Autodesk Fusion 360 part; units mm, degrees
note: some values were not read from the file. Chosen so that the rebuilt part matches the saved one: which bodies a step acts on. Set by a fixed rule: which sketch regions a step uses.
(part 4 of 6)
sketch "Sketch81" plane through (0, 0, 40) normal (0, 0, 1) x (-1, 0, 0)
  line L0 (-4, -129.3333) -> (-4, -109.2593)
  line L1 (-4, -109.2593) -> (-0.5, -109.2593)
  line L2 (-0.5, -109.2593) -> (-0.5, -90.7407)
  line L3 (-0.5, -90.7407) -> (-4, -90.7407)
  line L4 (-4, -90.7407) -> (-4, -70.6667)
  line L5 (-4, -70.6667) -> (-24.0741, -70.6667)
  line L6 (-24.0741, -70.6667) -> (-24.0741, -67.1667)
  line L7 (-24.0741, -67.1667) -> (-42.5926, -67.1667)
  line L8 (-42.5926, -67.1667) -> (-42.5926, -70.6667)
  line L9 (-42.5926, -70.6667) -> (-62.6667, -70.6667)
  line L10 (-62.6667, -70.6667) -> (-62.6667, -90.7407)
  line L11 (-62.6667, -90.7407) -> (-66.1667, -90.7407)
  line L12 (-66.1667, -90.7407) -> (-66.1667, -109.2593)
  line L13 (-66.1667, -109.2593) -> (-62.6667, -109.2593)
  line L14 (-62.6667, -109.2593) -> (-62.6667, -129.3333)
  line L15 (-62.6667, -129.3333) -> (-42.5926, -129.3333)
  line L16 (-42.5926, -129.3333) -> (-42.5926, -132.8333)
  line L17 (-42.5926, -132.8333) -> (-24.0741, -132.8333)
  line L18 (-24.0741, -132.8333) -> (-24.0741, -129.3333)
  line L19 (-24.0741, -129.3333) -> (-4, -129.3333)
  line L20 (-4, -129.3333) -> (-24.0741, -129.3333)
  line L21 (-24.0741, -129.3333) -> (-24.0741, -128.3333)
  line L22 (-24.0741, -128.3333) -> (-4, -128.3333)
  line L23 (-4, -128.3333) -> (-4, -129.3333)
  line L24 (-4, -129.3333) -> (-5, -129.3333)
  line L25 (-5, -129.3333) -> (-5, -109.2593)
  line L26 (-5, -109.2593) -> (-4, -109.2593)
  line L27 (-4, -109.2593) -> (-4, -129.3333)
  line L28 (-4, -70.6667) -> (-5, -70.6667)
  line L29 (-5, -70.6667) -> (-5, -90.7407)
  line L30 (-5, -90.7407) -> (-4, -90.7407)
  line L31 (-4, -90.7407) -> (-4, -70.6667)
  line L32 (-4, -70.6667) -> (-24.0741, -70.6667)
  line L33 (-24.0741, -70.6667) -> (-24.0741, -71.6667)
  line L34 (-24.0741, -71.6667) -> (-4, -71.6667)
  line L35 (-4, -71.6667) -> (-4, -70.6667)
  line L36 (-62.6667, -70.6667) -> (-42.5926, -70.6667)
  line L37 (-42.5926, -70.6667) -> (-42.5926, -71.6667)
  line L38 (-42.5926, -71.6667) -> (-62.6667, -71.6667)
  line L39 (-62.6667, -71.6667) -> (-62.6667, -70.6667)
  line L40 (-62.6667, -70.6667) -> (-61.6667, -70.6667)
  line L41 (-61.6667, -70.6667) -> (-61.6667, -90.7407)
  line L42 (-61.6667, -90.7407) -> (-62.6667, -90.7407)
  line L43 (-62.6667, -90.7407) -> (-62.6667, -70.6667)
  line L44 (-62.6667, -129.3333) -> (-61.6667, -129.3333)
  line L45 (-61.6667, -129.3333) -> (-61.6667, -109.2593)
  line L46 (-61.6667, -109.2593) -> (-62.6667, -109.2593)
  line L47 (-62.6667, -109.2593) -> (-62.6667, -129.3333)
  line L48 (-62.6667, -129.3333) -> (-42.5926, -129.3333)
  line L49 (-42.5926, -129.3333) -> (-42.5926, -128.3333)
  line L50 (-42.5926, -128.3333) -> (-62.6667, -128.3333)
  line L51 (-62.6667, -128.3333) -> (-62.6667, -129.3333)
  dimension "d549" = 1
  dimension "d550" = 1
  dimension "d551" = 1
  dimension "d552" = 1
  dimension "d553" = 1
  dimension "d554" = 1
  dimension "d555" = 1
  dimension "d556" = 1
  dimension "d557" = 20.0741
  dimension "d558" = 20.0741
  dimension "d559" = 20.0741
  dimension "d560" = 20.0741
  dimension "d561" = 20.0741
  dimension "d562" = 20.0741
  dimension "d563" = 20.0741
  dimension "d564" = 20.0741
  constraint horizontal L20
  constraint vertical L21
  constraint horizontal L22
  constraint vertical L23
  constraint coincident L0.start L19.end
  constraint horizontal L24
  constraint vertical L25
  constraint horizontal L26
  constraint vertical L27
  constraint horizontal L28
  constraint vertical L29
  constraint horizontal L30
  constraint vertical L31
  constraint coincident L4.end L5.start
  constraint horizontal L32
  constraint vertical L33
  constraint horizontal L34
  constraint vertical L35
  constraint horizontal L36
  constraint vertical L37
  constraint horizontal L38
  constraint vertical L39
  constraint coincident L9.end L10.start
  constraint horizontal L40
  constraint vertical L41
  constraint horizontal L42
  constraint vertical L43
  constraint horizontal L44
  constraint vertical L45
  constraint horizontal L46
  constraint vertical L47
  constraint coincident L14.end L15.start
  constraint horizontal L48
  constraint vertical L49
  constraint horizontal L50
  constraint vertical L51
  measures "d549" distance of L18.end L21.end
  measures "d550" distance of L15.end L49.end
  measures "d551" distance of L45.end L13.end
  measures "d552" distance of L9.end L40.end
  measures "d553" distance of L8.end L37.end
  measures "d554" distance of L5.end L33.end
  measures "d555" distance of L29.end L3.end
  measures "d556" distance of L25.end L0.end
  measures "d557" distance of L9.end L10.end
  measures "d558" distance of L14.end L13.end
  measures "d559" distance of L24.end L25.end
  measures "d560" distance of L28.end L29.end
  measures "d561" distance of L4.end L5.end
  measures "d562" distance of L9.end L8.end
  measures "d563" distance of L49.end L50.end
  measures "d564" distance of L21.end L22.end
extrude "Extrude50" cut sketch "Sketch81" against normal blind 4 contours L0 L19 L20 L22 L23 L24 L25 L27 | L0 L22 L25 L26 L27 | L19 L20 L21 L22 L25 | L4 L29 L30 L31 L34 | L15 L45 L48 L49 L50 | L4 L5 L28 L29 L31 L32 L34 L35 | L14 L15 L44 L45 L47 L48 L50 L51 | L5 L29 L32 L33 L34 | L14 L45 L46 L47 L50 | L9 L36 L37 L38 L41 | L10 L38 L41 L42 L43 | L9 L10 L36 L38 L39 L40 L41 L43 bodies 16
sketch "Sketch82" plane through (0, 0, 40) normal (0, 0, 1) x (-1, 0, 0)
  line L0 (-129.3333, -129.3333) -> (-109.2593, -129.3333)
  line L1 (-109.2593, -129.3333) -> (-109.2593, -132.8333)
  line L2 (-109.2593, -132.8333) -> (-90.7407, -132.8333)
  line L3 (-90.7407, -132.8333) -> (-90.7407, -129.3333)
  line L4 (-90.7407, -129.3333) -> (-70.6667, -129.3333)
  line L5 (-70.6667, -129.3333) -> (-70.6667, -109.2593)
  line L6 (-70.6667, -109.2593) -> (-67.1667, -109.2593)
  line L7 (-67.1667, -109.2593) -> (-67.1667, -90.7407)
  line L8 (-67.1667, -90.7407) -> (-70.6667, -90.7407)
  line L9 (-70.6667, -90.7407) -> (-70.6667, -70.6667)
  line L10 (-70.6667, -70.6667) -> (-90.7407, -70.6667)
  line L11 (-90.7407, -70.6667) -> (-90.7407, -67.1667)
  line L12 (-90.7407, -67.1667) -> (-109.2593, -67.1667)
  line L13 (-109.2593, -67.1667) -> (-109.2593, -70.6667)
  line L14 (-109.2593, -70.6667) -> (-129.3333, -70.6667)
  line L15 (-129.3333, -70.6667) -> (-129.3333, -90.7407)
  line L16 (-129.3333, -90.7407) -> (-132.8333, -90.7407)
  line L17 (-132.8333, -90.7407) -> (-132.8333, -109.2593)
  line L18 (-132.8333, -109.2593) -> (-129.3333, -109.2593)
  line L19 (-129.3333, -109.2593) -> (-129.3333, -129.3333)
  line L20 (-70.6667, -129.3333) -> (-90.7407, -129.3333)
  line L21 (-90.7407, -129.3333) -> (-90.7407, -128.3333)
  line L22 (-90.7407, -128.3333) -> (-70.6667, -128.3333)
  line L23 (-70.6667, -128.3333) -> (-70.6667, -129.3333)
  line L24 (-70.6667, -129.3333) -> (-71.6667, -129.3333)
  line L25 (-71.6667, -129.3333) -> (-71.6667, -109.2593)
  line L26 (-71.6667, -109.2593) -> (-70.6667, -109.2593)
  line L27 (-70.6667, -109.2593) -> (-70.6667, -129.3333)
  line L28 (-70.6667, -70.6667) -> (-71.6667, -70.6667)
  line L29 (-71.6667, -70.6667) -> (-71.6667, -90.7407)
  line L30 (-71.6667, -90.7407) -> (-70.6667, -90.7407)
  line L31 (-70.6667, -90.7407) -> (-70.6667, -70.6667)
  line L32 (-70.6667, -70.6667) -> (-90.7407, -70.6667)
  line L33 (-90.7407, -70.6667) -> (-90.7407, -71.6667)
  line L34 (-90.7407, -71.6667) -> (-70.6667, -71.6667)
  line L35 (-70.6667, -71.6667) -> (-70.6667, -70.6667)
  line L36 (-129.3333, -70.6667) -> (-109.2593, -70.6667)
  line L37 (-109.2593, -70.6667) -> (-109.2593, -71.6667)
  line L38 (-109.2593, -71.6667) -> (-129.3333, -71.6667)
  line L39 (-129.3333, -71.6667) -> (-129.3333, -70.6667)
  line L40 (-129.3333, -70.6667) -> (-128.3333, -70.6667)
  line L41 (-128.3333, -70.6667) -> (-128.3333, -90.7407)
  line L42 (-128.3333, -90.7407) -> (-129.3333, -90.7407)
  line L43 (-129.3333, -90.7407) -> (-129.3333, -70.6667)
  line L44 (-129.3333, -129.3333) -> (-128.3333, -129.3333)
  line L45 (-128.3333, -129.3333) -> (-128.3333, -109.2593)
  line L46 (-128.3333, -109.2593) -> (-129.3333, -109.2593)
  line L47 (-129.3333, -109.2593) -> (-129.3333, -129.3333)
  line L48 (-129.3333, -129.3333) -> (-109.2593, -129.3333)
  line L49 (-109.2593, -129.3333) -> (-109.2593, -128.3333)
  line L50 (-109.2593, -128.3333) -> (-129.3333, -128.3333)
  line L51 (-129.3333, -128.3333) -> (-129.3333, -129.3333)
  dimension "d567" = 1
  dimension "d568" = 1
  dimension "d569" = 1
  dimension "d570" = 1
  dimension "d571" = 1
  dimension "d572" = 1
  dimension "d573" = 1
  dimension "d574" = 1
  dimension "d575" = 20.0741
  dimension "d576" = 20.0741
  dimension "d577" = 20.0741
  dimension "d578" = 20.0741
  dimension "d579" = 20.0741
  dimension "d580" = 20.0741
  dimension "d581" = 20.0741
  dimension "d582" = 20.0741
  constraint horizontal L20
  constraint vertical L21
  constraint horizontal L22
  constraint vertical L23
  constraint coincident L4.end L5.start
  constraint horizontal L24
  constraint vertical L25
  constraint horizontal L26
  constraint vertical L27
  constraint horizontal L28
  constraint vertical L29
  constraint horizontal L30
  constraint vertical L31
  constraint coincident L9.end L10.start
  constraint horizontal L32
  constraint vertical L33
  constraint horizontal L34
  constraint vertical L35
  constraint horizontal L36
  constraint vertical L37
  constraint horizontal L38
  constraint vertical L39
  constraint coincident L14.end L15.start
  constraint horizontal L40
  constraint vertical L41
  constraint horizontal L42
  constraint vertical L43
  constraint horizontal L44
  constraint vertical L45
  constraint horizontal L46
  constraint vertical L47
  constraint coincident L0.start L19.end
  constraint horizontal L48
  constraint vertical L49
  constraint horizontal L50
  constraint vertical L51
  measures "d567" distance of L3.end L21.end
  measures "d568" distance of L0.end L49.end
  measures "d569" distance of L45.end L18.end
  measures "d570" distance of L41.end L15.end
  measures "d571" distance of L13.end L37.end
  measures "d572" distance of L10.end L33.end
  measures "d573" distance of L29.end L8.end
  measures "d574" distance of L25.end L5.end
  measures "d575" distance of L21.end L22.end
  measures "d576" distance of L49.end L50.end
  measures "d577" distance of L14.end L13.end
  measures "d578" distance of L9.end L10.end
  measures "d579" distance of L24.end L25.end
  measures "d580" distance of L44.end L45.end
  measures "d581" distance of L14.end L15.end
  measures "d582" distance of L9.end L8.end
extrude "Extrude51" cut sketch "Sketch82" against normal blind 4 contours L0 L19 L44 L45 L47 L48 L50 L51 | L0 L45 L48 L49 L50 | L19 L45 L46 L47 L50 | L4 L20 L21 L22 L25 | L15 L38 L41 L42 L43 | L4 L5 L20 L22 L23 L24 L25 L27 | L14 L15 L36 L38 L39 L40 L41 L43 | L5 L22 L25 L26 L27 | L14 L36 L37 L38 L41 | L9 L29 L30 L31 L34 | L10 L29 L32 L33 L34 | L9 L10 L28 L29 L31 L32 L34 L35 bodies 17
sketch "Sketch83" plane through (0, 0, 40) normal (0, 0, 1) x (-1, 0, 0)
  line L0 (-157.4074, -129.3333) -> (-137.3333, -129.3333)
  line L1 (-137.3333, -129.3333) -> (-137.3333, -109.2593)
  line L2 (-137.3333, -109.2593) -> (-133.8333, -109.2593)
  line L3 (-133.8333, -109.2593) -> (-133.8333, -90.7407)
  line L4 (-133.8333, -90.7407) -> (-137.3333, -90.7407)
  line L5 (-137.3333, -90.7407) -> (-137.3333, -70.6667)
  line L6 (-137.3333, -70.6667) -> (-157.4074, -70.6667)
  line L7 (-157.4074, -70.6667) -> (-157.4074, -67.1667)
  line L8 (-157.4074, -67.1667) -> (-175.9259, -67.1667)
  line L9 (-175.9259, -67.1667) -> (-175.9259, -70.6667)
  line L10 (-175.9259, -70.6667) -> (-196, -70.6667)
  line L11 (-196, -70.6667) -> (-196, -90.7407)
  line L12 (-196, -90.7407) -> (-199.5, -90.7407)
  line L13 (-199.5, -90.7407) -> (-199.5, -109.2593)
  line L14 (-199.5, -109.2593) -> (-196, -109.2593)
  line L15 (-196, -109.2593) -> (-196, -129.3333)
  line L16 (-196, -129.3333) -> (-175.9259, -129.3333)
  line L17 (-175.9259, -129.3333) -> (-175.9259, -132.8333)
  line L18 (-175.9259, -132.8333) -> (-157.4074, -132.8333)
  line L19 (-157.4074, -132.8333) -> (-157.4074, -129.3333)
  line L20 (-137.3333, -129.3333) -> (-157.4074, -129.3333)
  line L21 (-157.4074, -129.3333) -> (-157.4074, -128.3333)
  line L22 (-157.4074, -128.3333) -> (-137.3333, -128.3333)
  line L23 (-137.3333, -128.3333) -> (-137.3333, -129.3333)
  line L24 (-137.3333, -129.3333) -> (-138.3333, -129.3333)
  line L25 (-138.3333, -129.3333) -> (-138.3333, -109.2593)
  line L26 (-138.3333, -109.2593) -> (-137.3333, -109.2593)
  line L27 (-137.3333, -109.2593) -> (-137.3333, -129.3333)
  line L28 (-196, -129.3333) -> (-195, -129.3333)
  line L29 (-195, -129.3333) -> (-195, -109.2593)
  line L30 (-195, -109.2593) -> (-196, -109.2593)
  line L31 (-196, -109.2593) -> (-196, -129.3333)
  line L32 (-196, -129.3333) -> (-175.9259, -129.3333)
  line L33 (-175.9259, -129.3333) -> (-175.9259, -128.3333)
  line L34 (-175.9259, -128.3333) -> (-196, -128.3333)
  line L35 (-196, -128.3333) -> (-196, -129.3333)
  line L36 (-196, -70.6667) -> (-195, -70.6667)
  line L37 (-195, -70.6667) -> (-195, -90.7407)
  line L38 (-195, -90.7407) -> (-196, -90.7407)
  line L39 (-196, -90.7407) -> (-196, -70.6667)
  line L40 (-196, -70.6667) -> (-175.9259, -70.6667)
  line L41 (-175.9259, -70.6667) -> (-175.9259, -71.6667)
  line L42 (-175.9259, -71.6667) -> (-196, -71.6667)
  line L43 (-196, -71.6667) -> (-196, -70.6667)
  line L44 (-137.3333, -70.6667) -> (-157.4074, -70.6667)
  line L45 (-157.4074, -70.6667) -> (-157.4074, -71.6667)
  line L46 (-157.4074, -71.6667) -> (-137.3333, -71.6667)
  line L47 (-137.3333, -71.6667) -> (-137.3333, -70.6667)
  line L48 (-137.3333, -70.6667) -> (-138.3333, -70.6667)
  line L49 (-138.3333, -70.6667) -> (-138.3333, -90.7407)
  line L50 (-138.3333, -90.7407) -> (-137.3333, -90.7407)
  line L51 (-137.3333, -90.7407) -> (-137.3333, -70.6667)
  dimension "d585" = 1
  dimension "d586" = 1
  dimension "d587" = 1
  dimension "d588" = 1
  dimension "d589" = 1
  dimension "d590" = 1
  dimension "d591" = 1
  dimension "d592" = 1
  dimension "d593" = 20.0741
  dimension "d594" = 20.0741
  dimension "d595" = 20.0741
  dimension "d596" = 20.0741
  dimension "d597" = 20.0741
  dimension "d598" = 20.0741
  dimension "d599" = 20.0741
  dimension "d600" = 20.0741
  constraint horizontal L20
  constraint vertical L21
  constraint horizontal L22
  constraint vertical L23
  constraint coincident L0.end L1.start
  constraint horizontal L24
  constraint vertical L25
  constraint horizontal L26
  constraint vertical L27
  constraint horizontal L28
  constraint vertical L29
  constraint horizontal L30
  constraint vertical L31
  constraint coincident L15.end L16.start
  constraint horizontal L32
  constraint vertical L33
  constraint horizontal L34
  constraint vertical L35
  constraint horizontal L36
  constraint vertical L37
  constraint horizontal L38
  constraint vertical L39
  constraint coincident L10.end L11.start
  constraint horizontal L40
  constraint vertical L41
  constraint horizontal L42
  constraint vertical L43
  constraint horizontal L44
  constraint vertical L45
  constraint horizontal L46
  constraint vertical L47
  constraint coincident L5.end L6.start
  constraint horizontal L48
  constraint vertical L49
  constraint horizontal L50
  constraint vertical L51
  measures "d585" distance of L25.end L1.end
  measures "d586" distance of L0.start L21.end
  measures "d587" distance of L16.end L33.end
  measures "d588" distance of L29.end L14.end
  measures "d589" distance of L37.end L11.end
  measures "d590" distance of L9.end L41.end
  measures "d591" distance of L6.end L45.end
  measures "d592" distance of L49.end L4.end
  measures "d593" distance of L21.end L22.end
  measures "d594" distance of L33.end L34.end
  measures "d595" distance of L28.end L29.end
  measures "d596" distance of L24.end L25.end
  measures "d597" distance of L5.end L6.end
  measures "d598" distance of L10.end L9.end
  measures "d599" distance of L10.end L11.end
  measures "d600" distance of L48.end L49.end
extrude "Extrude52" cut sketch "Sketch83" against normal blind 4 contours L0 L20 L21 L22 L25 | L0 L1 L20 L22 L23 L24 L25 L27 | L1 L22 L25 L26 L27 | L16 L29 L32 L33 L34 | L15 L16 L28 L29 L31 L32 L34 L35 | L15 L29 L30 L31 L34 | L5 L46 L49 L50 L51 | L5 L6 L44 L46 L47 L48 L49 L51 | L6 L44 L45 L46 L49 | L11 L37 L38 L39 L42 | L10 L11 L36 L37 L39 L40 L42 L43 | L10 L37 L40 L41 L42 bodies 18
sketch "Sketch84" plane through (0, 0, 40) normal (0, 0, 1) x (-1, 0, 0)
  line L0 (-4, -157.4074) -> (-4, -137.3333)
  line L1 (-4, -137.3333) -> (-24.0741, -137.3333)
  line L2 (-24.0741, -137.3333) -> (-24.0741, -133.8333)
  line L3 (-24.0741, -133.8333) -> (-42.5926, -133.8333)
  line L4 (-42.5926, -133.8333) -> (-42.5926, -137.3333)
  line L5 (-42.5926, -137.3333) -> (-62.6667, -137.3333)
  line L6 (-62.6667, -137.3333) -> (-62.6667, -157.4074)
  line L7 (-62.6667, -157.4074) -> (-66.1667, -157.4074)
  line L8 (-66.1667, -157.4074) -> (-66.1667, -175.9259)
  line L9 (-66.1667, -175.9259) -> (-62.6667, -175.9259)
  line L10 (-62.6667, -175.9259) -> (-62.6667, -196)
  line L11 (-62.6667, -196) -> (-42.5926, -196)
  line L12 (-42.5926, -196) -> (-42.5926, -199.5)
  line L13 (-42.5926, -199.5) -> (-24.0741, -199.5)
  line L14 (-24.0741, -199.5) -> (-24.0741, -196)
  line L15 (-24.0741, -196) -> (-4, -196)
  line L16 (-4, -196) -> (-4, -175.9259)
  line L17 (-4, -175.9259) -> (-0.5, -175.9259)
  line L18 (-0.5, -175.9259) -> (-0.5, -157.4074)
  line L19 (-0.5, -157.4074) -> (-4, -157.4074)
  line L20 (-4, -196) -> (-24.0741, -196)
  line L21 (-24.0741, -196) -> (-24.0741, -195)
  line L22 (-24.0741, -195) -> (-4, -195)
  line L23 (-4, -195) -> (-4, -196)
  line L24 (-4, -196) -> (-5, -196)
  line L25 (-5, -196) -> (-5, -175.9259)
  line L26 (-5, -175.9259) -> (-4, -175.9259)
  line L27 (-4, -175.9259) -> (-4, -196)
  line L28 (-4, -137.3333) -> (-5, -137.3333)
  line L29 (-5, -137.3333) -> (-5, -157.4074)
  line L30 (-5, -157.4074) -> (-4, -157.4074)
  line L31 (-4, -157.4074) -> (-4, -137.3333)
  line L32 (-4, -137.3333) -> (-24.0741, -137.3333)
  line L33 (-24.0741, -137.3333) -> (-24.0741, -138.3333)
  line L34 (-24.0741, -138.3333) -> (-4, -138.3333)
  line L35 (-4, -138.3333) -> (-4, -137.3333)
  line L36 (-62.6667, -137.3333) -> (-42.5926, -137.3333)
  line L37 (-42.5926, -137.3333) -> (-42.5926, -138.3333)
  line L38 (-42.5926, -138.3333) -> (-62.6667, -138.3333)
  line L39 (-62.6667, -138.3333) -> (-62.6667, -137.3333)
  line L40 (-62.6667, -137.3333) -> (-61.6667, -137.3333)
  line L41 (-61.6667, -137.3333) -> (-61.6667, -157.4074)
  line L42 (-61.6667, -157.4074) -> (-62.6667, -157.4074)
  line L43 (-62.6667, -157.4074) -> (-62.6667, -137.3333)
  line L44 (-62.6667, -196) -> (-61.6667, -196)
  line L45 (-61.6667, -196) -> (-61.6667, -175.9259)
  line L46 (-61.6667, -175.9259) -> (-62.6667, -175.9259)
  line L47 (-62.6667, -175.9259) -> (-62.6667, -196)
  line L48 (-62.6667, -196) -> (-42.5926, -196)
  line L49 (-42.5926, -196) -> (-42.5926, -195)
  line L50 (-42.5926, -195) -> (-62.6667, -195)
  line L51 (-62.6667, -195) -> (-62.6667, -196)
  dimension "d605" = 1
  dimension "d606" = 1
  dimension "d607" = 1
  dimension "d608" = 1
  dimension "d609" = 1
  dimension "d610" = 1
  dimension "d611" = 1
  dimension "d613" = 1
  dimension "d614" = 20.0741
  dimension "d615" = 20.0741
  dimension "d616" = 20.0741
  dimension "d617" = 20.0741
  dimension "d618" = 20.0741
  dimension "d619" = 20.0741
  dimension "d620" = 20.0741
  dimension "d621" = 20.0741
  constraint horizontal L20
  constraint vertical L21
  constraint horizontal L22
  constraint vertical L23
  constraint coincident L15.end L16.start
  constraint horizontal L24
  constraint vertical L25
  constraint horizontal L26
  constraint vertical L27
  constraint horizontal L28
  constraint vertical L29
  constraint horizontal L30
  constraint vertical L31
  constraint coincident L0.end L1.start
  constraint horizontal L32
  constraint vertical L33
  constraint horizontal L34
  constraint vertical L35
  constraint horizontal L36
  constraint vertical L37
  constraint horizontal L38
  constraint vertical L39
  constraint coincident L5.end L6.start
  constraint horizontal L40
  constraint vertical L41
  constraint horizontal L42
  constraint vertical L43
  constraint horizontal L44
  constraint vertical L45
  constraint horizontal L46
  constraint vertical L47
  constraint coincident L10.end L11.start
  constraint horizontal L48
  constraint vertical L49
  constraint horizontal L50
  constraint vertical L51
  measures "d605" distance of L45.end L9.end
  measures "d606" distance of L41.end L6.end
  measures "d607" distance of L25.end L16.end
  measures "d608" distance of L29.end L0.start
  measures "d609" distance of L1.end L33.end
  measures "d610" distance of L4.end L37.end
  measures "d611" distance of L14.end L21.end
  measures "d613" distance of L11.end L49.end
  measures "d614" distance of L49.end L50.end
  measures "d615" distance of L21.end L22.end
  measures "d616" distance of L37.end L38.end
  measures "d617" distance of L33.end L34.end
  measures "d618" distance of L28.end L29.end
  measures "d619" distance of L24.end L25.end
  measures "d620" distance of L10.end L9.end
  measures "d621" distance of L5.end L6.end
extrude "Extrude53" cut sketch "Sketch84" against normal blind 4 contours L0 L29 L30 L31 L34 | L0 L1 L28 L29 L31 L32 L34 L35 | L1 L29 L32 L33 L34 | L16 L22 L25 L26 L27 | L15 L16 L20 L22 L23 L24 L25 L27 | L15 L20 L21 L22 L25 | L5 L36 L37 L38 L41 | L5 L6 L36 L38 L39 L40 L41 L43 | L6 L38 L41 L42 L43 | L11 L45 L48 L49 L50 | L10 L11 L44 L45 L47 L48 L50 L51 | L10 L45 L46 L47 L50 bodies 19
sketch "Sketch85" plane through (0, 0, 40) normal (0, 0, 1) x (-1, 0, 0)
  line L0 (-129.3333, -196) -> (-109.2593, -196)
  line L1 (-109.2593, -196) -> (-109.2593, -199.5)
  line L2 (-109.2593, -199.5) -> (-90.7407, -199.5)
  line L3 (-90.7407, -199.5) -> (-90.7407, -196)
  line L4 (-90.7407, -196) -> (-70.6667, -196)
  line L5 (-70.6667, -196) -> (-70.6667, -175.9259)
  line L6 (-70.6667, -175.9259) -> (-67.1667, -175.9259)
  line L7 (-67.1667, -175.9259) -> (-67.1667, -157.4074)
  line L8 (-67.1667, -157.4074) -> (-70.6667, -157.4074)
  line L9 (-70.6667, -157.4074) -> (-70.6667, -137.3333)
  line L10 (-70.6667, -137.3333) -> (-90.7407, -137.3333)
  line L11 (-90.7407, -137.3333) -> (-90.7407, -133.8333)
  line L12 (-90.7407, -133.8333) -> (-109.2593, -133.8333)
  line L13 (-109.2593, -133.8333) -> (-109.2593, -137.3333)
  line L14 (-109.2593, -137.3333) -> (-129.3333, -137.3333)
  line L15 (-129.3333, -137.3333) -> (-129.3333, -157.4074)
  line L16 (-129.3333, -157.4074) -> (-132.8333, -157.4074)
  line L17 (-132.8333, -157.4074) -> (-132.8333, -175.9259)
  line L18 (-132.8333, -175.9259) -> (-129.3333, -175.9259)
  line L19 (-129.3333, -175.9259) -> (-129.3333, -196)
  line L20 (-70.6667, -196) -> (-90.7407, -196)
  line L21 (-90.7407, -196) -> (-90.7407, -195)
  line L22 (-90.7407, -195) -> (-70.6667, -195)
  line L23 (-70.6667, -195) -> (-70.6667, -196)
  line L24 (-70.6667, -196) -> (-71.6667, -196)
  line L25 (-71.6667, -196) -> (-71.6667, -175.9259)
  line L26 (-71.6667, -175.9259) -> (-70.6667, -175.9259)
  line L27 (-70.6667, -175.9259) -> (-70.6667, -196)
  line L28 (-70.6667, -137.3333) -> (-71.6667, -137.3333)
  line L29 (-71.6667, -137.3333) -> (-71.6667, -157.4074)
  line L30 (-71.6667, -157.4074) -> (-70.6667, -157.4074)
  line L31 (-70.6667, -157.4074) -> (-70.6667, -137.3333)
  line L32 (-70.6667, -137.3333) -> (-90.7407, -137.3333)
  line L33 (-90.7407, -137.3333) -> (-90.7407, -138.3333)
  line L34 (-90.7407, -138.3333) -> (-70.6667, -138.3333)
  line L35 (-70.6667, -138.3333) -> (-70.6667, -137.3333)
  line L36 (-129.3333, -137.3333) -> (-109.2593, -137.3333)
  line L37 (-109.2593, -137.3333) -> (-109.2593, -138.3333)
  line L38 (-109.2593, -138.3333) -> (-129.3333, -138.3333)
  line L39 (-129.3333, -138.3333) -> (-129.3333, -137.3333)
  line L40 (-129.3333, -137.3333) -> (-128.3333, -137.3333)
  line L41 (-128.3333, -137.3333) -> (-128.3333, -157.4074)
  line L42 (-128.3333, -157.4074) -> (-129.3333, -157.4074)
  line L43 (-129.3333, -157.4074) -> (-129.3333, -137.3333)
  line L44 (-129.3333, -196) -> (-128.3333, -196)
  line L45 (-128.3333, -196) -> (-128.3333, -175.9259)
  line L46 (-128.3333, -175.9259) -> (-129.3333, -175.9259)
  line L47 (-129.3333, -175.9259) -> (-129.3333, -196)
  line L48 (-129.3333, -196) -> (-109.2593, -196)
  line L49 (-109.2593, -196) -> (-109.2593, -195)
  line L50 (-109.2593, -195) -> (-129.3333, -195)
  line L51 (-129.3333, -195) -> (-129.3333, -196)
  dimension "d624" = 1
  dimension "d625" = 1
  dimension "d626" = 1
  dimension "d627" = 1
  dimension "d628" = 1
  dimension "d629" = 1
  dimension "d630" = 1
  dimension "d631" = 1
  dimension "d632" = 20.0741
  dimension "d633" = 20.0741
  dimension "d634" = 20.0741
  dimension "d635" = 20.0741
  dimension "d636" = 20.0741
  dimension "d637" = 20.0741
  dimension "d638" = 20.0741
  dimension "d639" = 20.0741
  constraint horizontal L20
  constraint vertical L21
  constraint horizontal L22
  constraint vertical L23
  constraint coincident L4.end L5.start
  constraint horizontal L24
  constraint vertical L25
  constraint horizontal L26
  constraint vertical L27
  constraint horizontal L28
  constraint vertical L29
  constraint horizontal L30
  constraint vertical L31
  constraint coincident L9.end L10.start
  constraint horizontal L32
  constraint vertical L33
  constraint horizontal L34
  constraint vertical L35
  constraint horizontal L36
  constraint vertical L37
  constraint horizontal L38
  constraint vertical L39
  constraint coincident L14.end L15.start
  constraint horizontal L40
  constraint vertical L41
  constraint horizontal L42
  constraint vertical L43
  constraint horizontal L44
  constraint vertical L45
  constraint horizontal L46
  constraint vertical L47
  constraint coincident L0.start L19.end
  constraint horizontal L48
  constraint vertical L49
  constraint horizontal L50
  constraint vertical L51
  measures "d624" distance of L3.end L21.end
  measures "d625" distance of L0.end L49.end
  measures "d626" distance of L45.end L18.end
  measures "d627" distance of L41.end L15.end
  measures "d628" distance of L13.end L37.end
  measures "d629" distance of L10.end L33.end
  measures "d630" distance of L29.end L8.end
  measures "d631" distance of L25.end L5.end
  measures "d632" distance of L49.end L50.end
  measures "d633" distance of L21.end L22.end
  measures "d634" distance of L9.end L10.end
  measures "d635" distance of L14.end L13.end
  measures "d636" distance of L28.end L29.end
  measures "d637" distance of L24.end L25.end
  measures "d638" distance of L44.end L45.end
  measures "d639" distance of L14.end L15.end
extrude "Extrude54" cut sketch "Sketch85" against normal blind 4 contours L0 L19 L44 L45 L47 L48 L50 L51 | L0 L45 L48 L49 L50 | L19 L45 L46 L47 L50 | L4 L20 L21 L22 L25 | L15 L38 L41 L42 L43 | L4 L5 L20 L22 L23 L24 L25 L27 | L14 L15 L36 L38 L39 L40 L41 L43 | L5 L22 L25 L26 L27 | L14 L36 L37 L38 L41 | L9 L29 L30 L31 L34 | L10 L29 L32 L33 L34 | L9 L10 L28 L29 L31 L32 L34 L35 bodies 20
sketch "Sketch86" plane through (0, 0, 40) normal (0, 0, 1) x (-1, 0, 0)
  line L0 (-196, -196) -> (-175.9259, -196)
  line L1 (-175.9259, -196) -> (-175.9259, -199.5)
  line L2 (-175.9259, -199.5) -> (-157.4074, -199.5)
  line L3 (-157.4074, -199.5) -> (-157.4074, -196)
  line L4 (-157.4074, -196) -> (-137.3333, -196)
  line L5 (-137.3333, -196) -> (-137.3333, -175.9259)
  line L6 (-137.3333, -175.9259) -> (-133.8333, -175.9259)
  line L7 (-133.8333, -175.9259) -> (-133.8333, -157.4074)
  line L8 (-133.8333, -157.4074) -> (-137.3333, -157.4074)
  line L9 (-137.3333, -157.4074) -> (-137.3333, -137.3333)
  line L10 (-137.3333, -137.3333) -> (-157.4074, -137.3333)
  line L11 (-157.4074, -137.3333) -> (-157.4074, -133.8333)
  line L12 (-157.4074, -133.8333) -> (-175.9259, -133.8333)
  line L13 (-175.9259, -133.8333) -> (-175.9259, -137.3333)
  line L14 (-175.9259, -137.3333) -> (-196, -137.3333)
  line L15 (-196, -137.3333) -> (-196, -157.4074)
  line L16 (-196, -157.4074) -> (-199.5, -157.4074)
  line L17 (-199.5, -157.4074) -> (-199.5, -175.9259)
  line L18 (-199.5, -175.9259) -> (-196, -175.9259)
  line L19 (-196, -175.9259) -> (-196, -196)
  line L20 (-137.3333, -196) -> (-157.4074, -196)
  line L21 (-157.4074, -196) -> (-157.4074, -195)
  line L22 (-157.4074, -195) -> (-137.3333, -195)
  line L23 (-137.3333, -195) -> (-137.3333, -196)
  line L24 (-137.3333, -196) -> (-138.3333, -196)
  line L25 (-138.3333, -196) -> (-138.3333, -175.9259)
  line L26 (-138.3333, -175.9259) -> (-137.3333, -175.9259)
  line L27 (-137.3333, -175.9259) -> (-137.3333, -196)
  line L28 (-137.3333, -137.3333) -> (-138.3333, -137.3333)
  line L29 (-138.3333, -137.3333) -> (-138.3333, -157.4074)
  line L30 (-138.3333, -157.4074) -> (-137.3333, -157.4074)
  line L31 (-137.3333, -157.4074) -> (-137.3333, -137.3333)
  line L32 (-137.3333, -137.3333) -> (-157.4074, -137.3333)
  line L33 (-157.4074, -137.3333) -> (-157.4074, -138.3333)
  line L34 (-157.4074, -138.3333) -> (-137.3333, -138.3333)
  line L35 (-137.3333, -138.3333) -> (-137.3333, -137.3333)
  line L36 (-196, -137.3333) -> (-175.9259, -137.3333)
  line L37 (-175.9259, -137.3333) -> (-175.9259, -138.3333)
  line L38 (-175.9259, -138.3333) -> (-196, -138.3333)
  line L39 (-196, -138.3333) -> (-196, -137.3333)
  line L40 (-196, -137.3333) -> (-195, -137.3333)
  line L41 (-195, -137.3333) -> (-195, -157.4074)
  line L42 (-195, -157.4074) -> (-196, -157.4074)
  line L43 (-196, -157.4074) -> (-196, -137.3333)
  line L44 (-196, -196) -> (-195, -196)
  line L45 (-195, -196) -> (-195, -175.9259)
  line L46 (-195, -175.9259) -> (-196, -175.9259)
  line L47 (-196, -175.9259) -> (-196, -196)
  line L48 (-196, -196) -> (-175.9259, -196)
  line L49 (-175.9259, -196) -> (-175.9259, -195)
  line L50 (-175.9259, -195) -> (-196, -195)
  line L51 (-196, -195) -> (-196, -196)
  dimension "d642" = 1
  dimension "d643" = 1
  dimension "d644" = 1
  dimension "d645" = 1
  dimension "d646" = 1
  dimension "d647" = 1
  dimension "d648" = 1
  dimension "d649" = 1
  dimension "d650" = 20.0741
  dimension "d651" = 20.0741
  dimension "d652" = 20.0741
  dimension "d653" = 20.0741
  dimension "d654" = 20.0741
  dimension "d655" = 20.0741
  dimension "d656" = 20.0741
  dimension "d657" = 20.0741
  constraint horizontal L20
  constraint vertical L21
  constraint horizontal L22
  constraint vertical L23
  constraint coincident L4.end L5.start
  constraint horizontal L24
  constraint vertical L25
  constraint horizontal L26
  constraint vertical L27
  constraint horizontal L28
  constraint vertical L29
  constraint horizontal L30
  constraint vertical L31
  constraint coincident L9.end L10.start
  constraint horizontal L32
  constraint vertical L33
  constraint horizontal L34
  constraint vertical L35
  constraint horizontal L36
  constraint vertical L37
  constraint horizontal L38
  constraint vertical L39
  constraint coincident L14.end L15.start
  constraint horizontal L40
  constraint vertical L41
  constraint horizontal L42
  constraint vertical L43
  constraint horizontal L44
  constraint vertical L45
  constraint horizontal L46
  constraint vertical L47
  constraint coincident L0.start L19.end
  constraint horizontal L48
  constraint vertical L49
  constraint horizontal L50
  constraint vertical L51
  measures "d642" distance of L3.end L21.end
  measures "d643" distance of L0.end L49.end
  measures "d644" distance of L25.end L5.end
  measures "d645" distance of L45.end L18.end
  measures "d646" distance of L29.end L8.end
  measures "d647" distance of L10.end L33.end
  measures "d648" distance of L41.end L15.end
  measures "d649" distance of L13.end L37.end
  measures "d650" distance of L14.end L15.end
  measures "d651" distance of L28.end L29.end
  measures "d652" distance of L24.end L25.end
  measures "d653" distance of L44.end L45.end
  measures "d654" distance of L33.end L34.end
  measures "d655" distance of L37.end L38.end
  measures "d656" distance of L49.end L50.end
  measures "d657" distance of L21.end L22.end
extrude "Extrude55" cut sketch "Sketch86" against normal blind 4 contours L0 L19 L44 L45 L47 L48 L50 L51 | L0 L45 L48 L49 L50 | L19 L45 L46 L47 L50 | L4 L20 L21 L22 L25 | L15 L38 L41 L42 L43 | L4 L5 L20 L22 L23 L24 L25 L27 | L14 L15 L36 L38 L39 L40 L41 L43 | L5 L22 L25 L26 L27 | L14 L36 L37 L38 L41 | L9 L29 L30 L31 L34 | L10 L29 L32 L33 L34 | L9 L10 L28 L29 L31 L32 L34 L35 bodies 21
sketch "Hringur1" plane through (0, 0, 40) normal (0, 0, 1) x (-1, 0, 0)
  line L0 (-66.1667, -175.9259) -> (-61.6667, -175.9259)
  line L1 (-61.6667, -175.9259) -> (-61.6667, -195)
  line L2 (-61.6667, -195) -> (-42.5926, -195)
  line L3 (-42.5926, -195) -> (-42.5926, -199.5)
  line L4 (-42.5926, -199.5) -> (-24.0741, -199.5)
  line L5 (-24.0741, -199.5) -> (-24.0741, -195)
  line L6 (-24.0741, -195) -> (-5, -195)
  line L7 (-5, -195) -> (-5, -175.9259)
  line L8 (-5, -175.9259) -> (-0.5, -175.9259)
  line L9 (-0.5, -175.9259) -> (-0.5, -157.4074)
  line L10 (-0.5, -157.4074) -> (-5, -157.4074)
  line L11 (-5, -157.4074) -> (-5, -138.3333)
  line L12 (-5, -138.3333) -> (-24.0741, -138.3333)
  line L13 (-24.0741, -138.3333) -> (-24.0741, -133.8333)
  line L14 (-24.0741, -133.8333) -> (-42.5926, -133.8333)
  line L15 (-42.5926, -133.8333) -> (-42.5926, -138.3333)
  line L16 (-42.5926, -138.3333) -> (-61.6667, -138.3333)
  line L17 (-61.6667, -138.3333) -> (-61.6667, -157.4074)
  line L18 (-61.6667, -157.4074) -> (-66.1667, -157.4074)
  line L19 (-66.1667, -157.4074) -> (-66.1667, -175.9259)
  circle A0 centre (-33.3333, -166.6667) radius 16.4167
  circle A1 centre (-33.3333, -166.6667) radius 16.4167
  dimension "d665" = 32.8333
  dimension "d666" = 32.8333
  dimension "d667" = 32.8333
  dimension "d675" = 32.8333
  measures "d665" diameter of A0
  measures "d666" diameter of A1
  measures "d667" distance of L4 A0.centre
  measures "d675" distance of L19 A0.centre
extrude "Extrude56" cut sketch "Hringur1" against normal blind 4 contours A0 A1 bodies 19
sketch "Hringur2" plane through (0, 0, 40) normal (0, 0, 1) x (-1, 0, 0)
  line L0 (-67.1667, -157.4074) -> (-71.6667, -157.4074)
  line L1 (-71.6667, -157.4074) -> (-71.6667, -138.3333)
  line L2 (-71.6667, -138.3333) -> (-90.7407, -138.3333)
  line L3 (-90.7407, -138.3333) -> (-90.7407, -133.8333)
  line L4 (-90.7407, -133.8333) -> (-109.2593, -133.8333)
  line L5 (-109.2593, -133.8333) -> (-109.2593, -138.3333)
  line L6 (-109.2593, -138.3333) -> (-128.3333, -138.3333)
  line L7 (-128.3333, -138.3333) -> (-128.3333, -157.4074)
  line L8 (-128.3333, -157.4074) -> (-132.8333, -157.4074)
  line L9 (-132.8333, -157.4074) -> (-132.8333, -175.9259)
  line L10 (-132.8333, -175.9259) -> (-128.3333, -175.9259)
  line L11 (-128.3333, -175.9259) -> (-128.3333, -195)
  line L12 (-128.3333, -195) -> (-109.2593, -195)
  line L13 (-109.2593, -195) -> (-109.2593, -199.5)
  line L14 (-109.2593, -199.5) -> (-90.7407, -199.5)
  line L15 (-90.7407, -199.5) -> (-90.7407, -195)
  line L16 (-90.7407, -195) -> (-71.6667, -195)
  line L17 (-71.6667, -195) -> (-71.6667, -175.9259)
  line L18 (-71.6667, -175.9259) -> (-67.1667, -175.9259)
  line L19 (-67.1667, -175.9259) -> (-67.1667, -157.4074)
  circle A0 centre (-100, -166.6667) radius 16.4167
  dimension "d676" = 32.8333
  dimension "d684" = 32.8333
  dimension "d685" = 32.8333
  measures "d676" diameter of A0
  measures "d684" distance of L9 A0.centre
  measures "d685" distance of L14 A0.centre
extrude "Extrude58" cut sketch "Hringur2" against normal blind 4 contours A0 bodies 20
sketch "Hringur3" plane through (0, 0, 40) normal (0, 0, 1) x (-1, 0, 0)
  line L0 (-199.5, -175.9259) -> (-195, -175.9259)
  line L1 (-195, -175.9259) -> (-195, -195)
  line L2 (-195, -195) -> (-175.9259, -195)
  line L3 (-175.9259, -195) -> (-175.9259, -199.5)
  line L4 (-175.9259, -199.5) -> (-157.4074, -199.5)
  line L5 (-157.4074, -199.5) -> (-157.4074, -195)
  line L6 (-157.4074, -195) -> (-138.3333, -195)
  line L7 (-138.3333, -195) -> (-138.3333, -175.9259)
  line L8 (-138.3333, -175.9259) -> (-133.8333, -175.9259)
  line L9 (-133.8333, -175.9259) -> (-133.8333, -157.4074)
  line L10 (-133.8333, -157.4074) -> (-138.3333, -157.4074)
  line L11 (-138.3333, -157.4074) -> (-138.3333, -138.3333)
  line L12 (-138.3333, -138.3333) -> (-157.4074, -138.3333)
  line L13 (-157.4074, -138.3333) -> (-157.4074, -133.8333)
  line L14 (-157.4074, -133.8333) -> (-175.9259, -133.8333)
  line L15 (-175.9259, -133.8333) -> (-175.9259, -138.3333)
  line L16 (-175.9259, -138.3333) -> (-195, -138.3333)
  line L17 (-195, -138.3333) -> (-195, -157.4074)
  line L18 (-195, -157.4074) -> (-199.5, -157.4074)
  line L19 (-199.5, -157.4074) -> (-199.5, -175.9259)
  circle A0 centre (-166.6667, -166.6667) radius 16.4167
  dimension "d679" = 32.8333
  dimension "d680" = 32.8333
  dimension "d681" = 32.8333
  measures "d679" diameter of A0
  measures "d680" distance of L4 A0.centre
  measures "d681" distance of L19 A0.centre
extrude "Extrude59" cut sketch "Hringur3" against normal blind 4 contours A0 bodies 21
sketch "Hringur4" plane through (0, 0, 40) normal (0, 0, 1) x (-1, 0, 0)
  line L0 (-66.1667, -109.2593) -> (-61.6667, -109.2593)
  line L1 (-61.6667, -109.2593) -> (-61.6667, -128.3333)
  line L2 (-61.6667, -128.3333) -> (-42.5926, -128.3333)
  line L3 (-42.5926, -128.3333) -> (-42.5926, -132.8333)
  line L4 (-42.5926, -132.8333) -> (-24.0741, -132.8333)
  line L5 (-24.0741, -132.8333) -> (-24.0741, -128.3333)
  line L6 (-24.0741, -128.3333) -> (-5, -128.3333)
  line L7 (-5, -128.3333) -> (-5, -109.2593)
  line L8 (-5, -109.2593) -> (-0.5, -109.2593)
  line L9 (-0.5, -109.2593) -> (-0.5, -90.7407)
  line L10 (-0.5, -90.7407) -> (-5, -90.7407)
  line L11 (-5, -90.7407) -> (-5, -71.6667)
  line L12 (-5, -71.6667) -> (-24.0741, -71.6667)
  line L13 (-24.0741, -71.6667) -> (-24.0741, -67.1667)
  line L14 (-24.0741, -67.1667) -> (-42.5926, -67.1667)
  line L15 (-42.5926, -67.1667) -> (-42.5926, -71.6667)
  line L16 (-42.5926, -71.6667) -> (-61.6667, -71.6667)
  line L17 (-61.6667, -71.6667) -> (-61.6667, -90.7407)
  line L18 (-61.6667, -90.7407) -> (-66.1667, -90.7407)
  line L19 (-66.1667, -90.7407) -> (-66.1667, -109.2593)
  circle A0 centre (-33.3333, -100) radius 16.4167
  dimension "d686" = 32.8333
  dimension "d687" = 32.8333
  dimension "d688" = 32.8333
  measures "d686" diameter of A0
  measures "d687" distance of L19 A0.centre
  measures "d688" distance of L4 A0.centre
extrude "Extrude60" cut sketch "Hringur4" against normal blind 4 contours A0 bodies 16
sketch "Sketch93" plane through (0, 0, 40) normal (0, 0, 1) x (-1, 0, 0)
  line L0 (-67.1667, -90.7407) -> (-71.6667, -90.7407)
  line L1 (-71.6667, -90.7407) -> (-71.6667, -71.6667)
  line L2 (-71.6667, -71.6667) -> (-90.7407, -71.6667)
  line L3 (-90.7407, -71.6667) -> (-90.7407, -67.1667)
  line L4 (-90.7407, -67.1667) -> (-109.2593, -67.1667)
  line L5 (-109.2593, -67.1667) -> (-109.2593, -71.6667)
  line L6 (-109.2593, -71.6667) -> (-128.3333, -71.6667)
  line L7 (-128.3333, -71.6667) -> (-128.3333, -90.7407)
  line L8 (-128.3333, -90.7407) -> (-132.8333, -90.7407)
  line L9 (-132.8333, -90.7407) -> (-132.8333, -109.2593)
  line L10 (-132.8333, -109.2593) -> (-128.3333, -109.2593)
  line L11 (-128.3333, -109.2593) -> (-128.3333, -128.3333)
  line L12 (-128.3333, -128.3333) -> (-109.2593, -128.3333)
  line L13 (-109.2593, -128.3333) -> (-109.2593, -132.8333)
  line L14 (-109.2593, -132.8333) -> (-90.7407, -132.8333)
  line L15 (-90.7407, -132.8333) -> (-90.7407, -128.3333)
  line L16 (-90.7407, -128.3333) -> (-71.6667, -128.3333)
  line L17 (-71.6667, -128.3333) -> (-71.6667, -109.2593)
  line L18 (-71.6667, -109.2593) -> (-67.1667, -109.2593)
  line L19 (-67.1667, -109.2593) -> (-67.1667, -90.7407)
  line L20 (-87.6252, -112.3748) -> (-89.9469, -114.6964)
  line L21 (-89.9469, -114.6964) -> (-100, -104.6433)
  line L22 (-87.6252, -112.3748) -> (-85.3036, -110.0531)
  line L23 (-100, -104.6433) -> (-110.0531, -114.6964)
  line L24 (-110.0531, -114.6964) -> (-112.3748, -112.3748)
  line L25 (-112.3748, -112.3748) -> (-114.6964, -110.0531)
  line L26 (-114.6964, -110.0531) -> (-104.6433, -100)
  line L27 (-85.3036, -110.0531) -> (-95.3567, -100)
  line L28 (-85.3036, -89.9469) -> (-95.3567, -100)
  line L29 (-87.6252, -87.6252) -> (-85.3036, -89.9469)
  line L30 (-87.6252, -87.6252) -> (-89.9469, -85.3036)
  line L31 (-89.9469, -85.3036) -> (-100, -95.3567)
  line L32 (-100, -95.3567) -> (-110.0531, -85.3036)
  line L33 (-110.0531, -85.3036) -> (-112.3748, -87.6252)
  line L34 (-112.3748, -87.6252) -> (-114.6964, -89.9469)
  line L35 (-114.6964, -89.9469) -> (-104.6433, -100)
  dimension "d693" = 3.2833
  dimension "d694" = 3.2833
  dimension "d695" = 14.2173
  dimension "d696" = 14.2173
  dimension "d697" = 3.2833
  dimension "d698" = 3.2833
  dimension "d701" = 28.19
  dimension "d702" = 28.19
  constraint perpendicular L20 L21
  constraint perpendicular L21 L23
  constraint perpendicular L25 L26
  constraint perpendicular L22 L27
  measures "d693" distance of L20.start L20.end
  measures "d694" distance of L20.start L22.end
  measures "d695" distance of L20.end L21.end
  measures "d696" distance of L21.end L23.end
  measures "d697" distance of L23.end L24.end
  measures "d698" distance of L24.end L25.end
  measures "d701" distance of L9 L26.end
  measures "d702" distance of L14 L21.end
sketch "Sketch95" plane through (0, 0, 40) normal (0, 0, 1) x (-1, 0, 0)
  line L0 (-175.9259, -67.1667) -> (-175.9259, -71.6667)
  line L1 (-175.9259, -71.6667) -> (-195, -71.6667)
  line L2 (-195, -71.6667) -> (-195, -90.7407)
  line L3 (-195, -90.7407) -> (-199.5, -90.7407)
  line L4 (-199.5, -90.7407) -> (-199.5, -109.2593)
  line L5 (-199.5, -109.2593) -> (-195, -109.2593)
  line L6 (-195, -109.2593) -> (-195, -128.3333)
  line L7 (-195, -128.3333) -> (-175.9259, -128.3333)
  line L8 (-175.9259, -128.3333) -> (-175.9259, -132.8333)
  line L9 (-175.9259, -132.8333) -> (-157.4074, -132.8333)
  line L10 (-157.4074, -132.8333) -> (-157.4074, -128.3333)
  line L11 (-157.4074, -128.3333) -> (-138.3333, -128.3333)
  line L12 (-138.3333, -128.3333) -> (-138.3333, -109.2593)
  line L13 (-138.3333, -109.2593) -> (-133.8333, -109.2593)
  line L14 (-133.8333, -109.2593) -> (-133.8333, -90.7407)
  line L15 (-133.8333, -90.7407) -> (-138.3333, -90.7407)
  line L16 (-138.3333, -90.7407) -> (-138.3333, -71.6667)
  line L17 (-138.3333, -71.6667) -> (-157.4074, -71.6667)
  line L18 (-157.4074, -71.6667) -> (-157.4074, -67.1667)
  line L19 (-157.4074, -67.1667) -> (-175.9259, -67.1667)
  line L20 (-154.2919, -87.6252) -> (-151.9702, -89.9469)
  line L21 (-154.2919, -112.3748) -> (-151.9702, -110.0531)
  line L22 (-154.2919, -112.3748) -> (-156.6136, -114.6964)
  line L23 (-156.6136, -114.6964) -> (-166.6667, -104.6433)
  line L24 (-154.2919, -87.6252) -> (-156.6136, -85.3036)
  line L25 (-151.9702, -110.0531) -> (-162.0233, -100)
  line L26 (-176.7198, -114.6964) -> (-179.0414, -112.3748)
  line L27 (-176.7198, -85.3036) -> (-179.0414, -87.6252)
  line L28 (-166.6667, -95.3567) -> (-176.7198, -85.3036)
  line L29 (-166.6667, -104.6433) -> (-176.7198, -114.6964)
  line L30 (-181.3631, -110.0531) -> (-171.31, -100)
  line L31 (-151.9702, -89.9469) -> (-162.0233, -100)
  line L32 (-156.6136, -85.3036) -> (-166.6667, -95.3567)
  line L33 (-181.3631, -89.9469) -> (-171.31, -100)
  line L34 (-179.0414, -87.6252) -> (-181.3631, -89.9469)
  line L35 (-179.0414, -112.3748) -> (-181.3631, -110.0531)
  dimension "d703" = 3.2833
  dimension "d704" = 3.2833
  dimension "d705" = 14.2173
  dimension "d706" = 14.2173
  dimension "d707" = 3.2833
  dimension "d708" = 3.2833
  constraint perpendicular L22 L23
  constraint perpendicular L23 L29
  constraint perpendicular L30 L35
  constraint perpendicular L21 L25
  measures "d703" distance of L22.end L21.start
  measures "d704" distance of L21.end L21.start
  measures "d705" distance of L23.end L22.end
  measures "d706" distance of L26.start L23.end
  measures "d707" distance of L26.start L26.end
  measures "d708" distance of L26.end L30.start
sketch "Sketch96" plane through (0, 0, 40) normal (0, 0, 1) x (-1, 0, 0)
  line L0 (-157.4074, -66.1667) -> (-157.4074, -61.6667)
  line L1 (-157.4074, -61.6667) -> (-138.3333, -61.6667)
  line L2 (-138.3333, -61.6667) -> (-138.3333, -42.5926)
  line L3 (-138.3333, -42.5926) -> (-133.8333, -42.5926)
  line L4 (-133.8333, -42.5926) -> (-133.8333, -24.0741)
  line L5 (-133.8333, -24.0741) -> (-138.3333, -24.0741)
  line L6 (-138.3333, -24.0741) -> (-138.3333, -5)
  line L7 (-138.3333, -5) -> (-157.4074, -5)
  line L8 (-157.4074, -5) -> (-157.4074, -0.5)
  line L9 (-157.4074, -0.5) -> (-175.9259, -0.5)
  line L10 (-175.9259, -0.5) -> (-175.9259, -5)
  line L11 (-175.9259, -5) -> (-195, -5)
  line L12 (-195, -5) -> (-195, -24.0741)
  line L13 (-195, -24.0741) -> (-199.5, -24.0741)
  line L14 (-199.5, -24.0741) -> (-199.5, -42.5926)
  line L15 (-199.5, -42.5926) -> (-195, -42.5926)
  line L16 (-195, -42.5926) -> (-195, -61.6667)
  line L17 (-195, -61.6667) -> (-175.9259, -61.6667)
  line L18 (-175.9259, -61.6667) -> (-175.9259, -66.1667)
  line L19 (-175.9259, -66.1667) -> (-157.4074, -66.1667)
  line L20 (-176.7198, -48.0298) -> (-179.0414, -45.7081)
  line L21 (-181.3631, -43.3864) -> (-171.31, -33.3333)
  line L22 (-156.6136, -48.0298) -> (-166.6667, -37.9767)
  line L23 (-154.2919, -45.7081) -> (-156.6136, -48.0298)
  line L24 (-151.9702, -43.3864) -> (-162.0233, -33.3333)
  line L25 (-179.0414, -45.7081) -> (-181.3631, -43.3864)
  line L26 (-156.6136, -18.6369) -> (-166.6667, -28.69)
  line L27 (-154.2919, -20.9586) -> (-156.6136, -18.6369)
  line L28 (-176.7198, -18.6369) -> (-179.0414, -20.9586)
  line L29 (-181.3631, -23.2802) -> (-171.31, -33.3333)
  line L30 (-179.0414, -20.9586) -> (-181.3631, -23.2802)
  line L31 (-166.6667, -28.69) -> (-176.7198, -18.6369)
  line L32 (-151.9702, -23.2802) -> (-162.0233, -33.3333)
  line L33 (-166.6667, -37.9767) -> (-176.7198, -48.0298)
  line L34 (-154.2919, -45.7081) -> (-151.9702, -43.3864)
  line L35 (-154.2919, -20.9586) -> (-151.9702, -23.2802)
  dimension "d709" = 3.2833
  dimension "d710" = 3.2833
  dimension "d711" = 14.2173
  dimension "d712" = 14.2173
  dimension "d713" = 3.2833
  dimension "d714" = 3.2833
  constraint perpendicular L22 L23
  constraint perpendicular L22 L33
  constraint perpendicular L21 L25
  constraint perpendicular L24 L34
  measures "d709" distance of L22.start L23.start
  measures "d710" distance of L23.start L24.start
  measures "d711" distance of L22.start L22.end
  measures "d712" distance of L20.start L22.end
  measures "d713" distance of L20.start L20.end
  measures "d714" distance of L20.end L21.start
sketch "Sketch97" plane through (0, 0, 40) normal (0, 0, 1) x (-1, 0, 0)
  line L0 (-67.1667, -24.0741) -> (-71.6667, -24.0741)
  line L1 (-71.6667, -24.0741) -> (-71.6667, -5)
  line L2 (-71.6667, -5) -> (-90.7407, -5)
  line L3 (-90.7407, -5) -> (-90.7407, -0.5)
  line L4 (-90.7407, -0.5) -> (-109.2593, -0.5)
  line L5 (-109.2593, -0.5) -> (-109.2593, -5)
  line L6 (-109.2593, -5) -> (-128.3333, -5)
  line L7 (-128.3333, -5) -> (-128.3333, -24.0741)
  line L8 (-128.3333, -24.0741) -> (-132.8333, -24.0741)
  line L9 (-132.8333, -24.0741) -> (-132.8333, -42.5926)
  line L10 (-132.8333, -42.5926) -> (-128.3333, -42.5926)
  line L11 (-128.3333, -42.5926) -> (-128.3333, -61.6667)
  line L12 (-128.3333, -61.6667) -> (-109.2593, -61.6667)
  line L13 (-109.2593, -61.6667) -> (-109.2593, -66.1667)
  line L14 (-109.2593, -66.1667) -> (-90.7407, -66.1667)
  line L15 (-90.7407, -66.1667) -> (-90.7407, -61.6667)
  line L16 (-90.7407, -61.6667) -> (-71.6667, -61.6667)
  line L17 (-71.6667, -61.6667) -> (-71.6667, -42.5926)
  line L18 (-71.6667, -42.5926) -> (-67.1667, -42.5926)
  line L19 (-67.1667, -42.5926) -> (-67.1667, -24.0741)
  line L20 (-87.6252, -20.9586) -> (-89.9469, -18.6369)
  line L21 (-100, -28.69) -> (-110.0531, -18.6369)
  line L22 (-87.6252, -45.7081) -> (-89.9469, -48.0298)
  line L23 (-112.3748, -20.9586) -> (-114.6964, -23.2802)
  line L24 (-112.3748, -45.7081) -> (-114.6964, -43.3864)
  line L25 (-114.6964, -43.3864) -> (-104.6433, -33.3333)
  line L26 (-110.0531, -18.6369) -> (-112.3748, -20.9586)
  line L27 (-110.0531, -48.0298) -> (-112.3748, -45.7081)
  line L28 (-100, -37.9767) -> (-110.0531, -48.0298)
  line L29 (-85.3036, -43.3864) -> (-95.3567, -33.3333)
  line L30 (-114.6964, -23.2802) -> (-104.6433, -33.3333)
  line L31 (-89.9469, -48.0298) -> (-100, -37.9767)
  line L32 (-87.6252, -20.9586) -> (-85.3036, -23.2802)
  line L33 (-89.9469, -18.6369) -> (-100, -28.69)
  line L34 (-87.6252, -45.7081) -> (-85.3036, -43.3864)
  line L35 (-85.3036, -23.2802) -> (-95.3567, -33.3333)
  dimension "d715" = 3.2833
  dimension "d716" = 3.2833
  dimension "d717" = 14.2173
  dimension "d718" = 14.2173
  dimension "d719" = 3.2833
  dimension "d720" = 3.2833
  constraint perpendicular L22 L31
  constraint perpendicular L28 L31
  constraint perpendicular L24 L25
  constraint perpendicular L29 L34
  measures "d715" distance of L22.start L22.end
  measures "d716" distance of L29.start L22.start
  measures "d717" distance of L22.end L28.start
  measures "d718" distance of L27.start L28.start
  measures "d719" distance of L27.start L24.start
  measures "d720" distance of L24.start L24.end